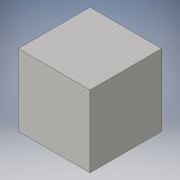
# Autodesk Inventor part: C
Saved by Autodesk Inventor 2016 (Build 200138000, 138)
## iProperties
Created: 2015-10-29
Part Number: C
Material: Generic
Document SubType Name: Modeling
Designer: nightstalker
Density: 1 g/cm^3
Appearance: Default
Mass: 27 g
Surface Area: 54 cm^2
Volume: 27 cm^3
Author: nightstalker
Autodesk Inventor part; units mm, degrees
ref_plane "YZ Plane" through (0, 0, 0) normal (1, 0, 0) x (0, 1, 0)
ref_plane "XZ Plane" through (0, 0, 0) normal (0, 1, 0) x (-1, 0, 0)
ref_plane "XY Plane" through (0, 0, 0) normal (0, 0, 1) x (1, 0, 0)
sketch "Sketch1" plane through (0, 0, 0) normal (0, 1, 0) x (-1, 0, 0)
  line L0 (0, 0) -> (-30, 0)
  line L1 (-30, 0) -> (-30, -30)
  line L2 (-30, -30) -> (0, -30)
  line L3 (0, -30) -> (0, 0)
  dimension "d0" = 30
  dimension "d1" = 30
  constraints: 8 end point, 2 parallel, 1 horizontal, 1 perpendicular
  measures "d0" distance of L2.end L1.end
  measures "d1" distance of L1.end L0.end
extrude "Extrusion1" add sketch "Sketch1" along normal blind 30
body "Solid1"
